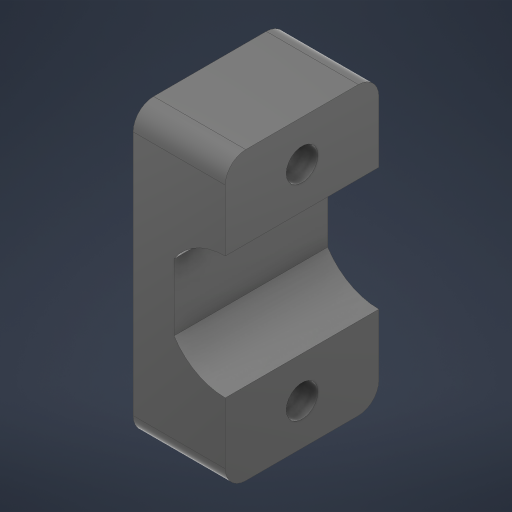
# Autodesk Inventor part: podstawka silnika
Saved by Autodesk Inventor 2024 (Build 280153000, 153)
## iProperties
Created: 2024-05-23
Part Number: podstawka silnika
Material: ABS Plastic
Document SubType Name: Modeling
Designer: Adam
Density: 1.06 g/cm^3
Appearance: Smooth - White
Mass: 3.00489 g
Surface Area: 17.1369 cm^2
Volume: 2.8348 cm^3
Author: Adam
Autodesk Inventor part; units mm, degrees
ref_plane "YZ Plane" through (0, 0, 0) normal (1, 0, 0) x (0, 1, 0)
ref_plane "XZ Plane" through (0, 0, 0) normal (0, 1, 0) x (-1, 0, 0)
sketch "Sketch2" plane through (0, 0, 0) normal (0, 0, 1) x (1, 0, 0)
  line L0 (3.1675, -3.2086) -> (3.1675, 0.0414)
  arc A0 (8.1675, 2.7916) -> (3.1675, 0.0414) centre (8.1675, -3.1285) ccw
  line L1 (5.3308, -15.8516) -> (5.3308, -15.8516)
  line L2 (8.1675, 2.7916) -> (8.1675, 10.7916)
  line L3 (3.1675, -3.2086) -> (3.1675, -6.4586)
  arc A1 (3.1675, -6.4586) -> (8.1675, -9.2089) centre (8.1675, -3.2888) ccw
  line L4 (8.1675, -9.2089) -> (8.1675, -17.2089)
  line L5 (8.1675, 10.7916) -> (-0.8325, 10.7916)
  line L6 (8.1675, -17.2089) -> (-0.8325, -17.2089)
  line L7 (-0.8325, 10.7916) -> (-0.8325, -17.2089)
  point P0 (0, 0)
  point P1 (8.1675, -9.2089)
  dimension "d10" = 9
  dimension "d11" = 4
  constraints: 16 end point, 4 point on circle, 2 centre point, 2 horizontal, 1 perpendicular
  measures "d10" distance between parallel lines of L7 L4
  measures "d11" distance between parallel lines of L7 L3
extrude "Extrusion2" add sketch "Sketch2" along normal blind 15
ref_plane "Work Plane1" through (-0.8325, -3.2086, 0) normal (0, 1, 0) x (1, 0, 0)
sketch "Sketch3" plane through (-0.8325, -17.2089, 0) normal (-1, 0, 0) x (0, 0, 1)
  line L0 (0, 28.0006) -> (0, 0) projected
  line L1 (0, 0) -> (15, 0) projected
  line L2 (0, 28.0006) -> (15, 28.0006) projected
  point P0 (7.5, 4)
  point P1 (7.5, 24.0006)
  point P2 (7.5, 0)
  point P3 (7.5, 28.0006)
  dimension "d16" = 7.5
  dimension "d17" = 4
  dimension "d18" = 4
  dimension "d19" = 7.5
  constraints: 2 midpoint
  measures "d16" distance from line of L0 point (7.5, 4)
  measures "d17" distance of point (7.5, 0) point (7.5, 4)
  measures "d18" distance of point (7.5, 28.001) point (7.5, 24.001)
  measures "d19" distance from line of L0 point (7.5, 24.001)
hole "Hole1" at (-0.8325, -13.2089, 7.5) at (-0.8325, 6.7916, 7.5) direction (1, 0, 0) diameter 3.1 end through all
fillet "Fillet1" radius 2 4 edges at (3.6675, 10.7916, 15) (3.6675, 10.7916, 0) (3.6675, -17.2089, 0) (3.6675, -17.2089, 15)
body "Solid2"
